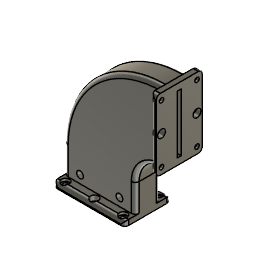
Receiver (Autodesk Fusion 360 design; units mm, degrees)
Autodesk Fusion 360 part; units mm, degrees
sketch "Sketch1" plane through (0, 0, 0) normal (0, 1, 0) x (1, 0, 0)
  circle A0 centre (69, 0) radius 69
  circle A1 centre (69, 0) radius 25
  circle A2 centre (45.471119, -40.686506) radius 22 construction
  line L0 (0, 15) -> (44, 15) construction
  circle A3 centre (37, 15) radius 2.6
  line L1 (22, 15) -> (22, 6) construction
  circle A4 centre (7, 15) radius 2.6
  line L2 (0, 0) -> (0, 25)
  line L3 (0, 25) -> (44, 25)
  line L4 (44, 25) -> (44, 0)
  line L5 (69, -25) -> (69, -69)
  dimension "d1" = 44
  dimension "d2" = 5.2
  dimension "d3" = 15
  dimension "d4" = 25
  dimension "d5" = 50
  dimension "d6" = 10
  constraint coincident L2.start A0
  constraint concentric A0 A1
  constraint tangent A1 A2
  constraint tangent A0 A2
  constraint horizontal L2.start A0.centre
  constraint horizontal L0
  constraint coincident L0 A3.centre
  constraint midpoint L0 L1.start
  constraint perpendicular L0 L1
  constraint symmetric A3 L1 A4
  constraint tangent A0 L2
  constraint perpendicular L0 L2
  constraint perpendicular L2 L3
  constraint perpendicular L3 L4
  constraint coincident L2.start origin
  constraint coincident L4 L0.end
  constraint coincident A1 L4.end
  constraint horizontal A0.centre L4.end
  constraint coincident L0.start L2
  constraint coincident A1 L5.start
  constraint coincident A0 L5.end
  constraint vertical L5
  constraint vertical A0.centre L5.start
  measures "d1" diameter of A2
  measures "d2" diameter of A3
  measures "d3" distance of A3.centre L1
  measures "d4" distance of L2.start L2.end
  measures "d5" diameter of A1
  measures "d6" distance of A3.centre L3
extrude "Extrude1" add sketch "Sketch1" along normal blind 8 contours A0 A1 L3 L4 L5 | A0 L2 L3 picked at (26.77857, -0.136786) picked at (2.261752, 22.293862)
sketch "Sketch2" plane through (0, 8, 0) normal (0, 1, 0) x (-1, 0, 0)
  circle A0 centre (-7, -15) radius 2.6
  circle A1 centre (-37, -15) radius 2.6
  arc A2 (0, 0) -> (-69, 69) centre (-69, 0) ccw
  line L0 (-69, 69) -> (-69, 25)
  arc A3 (-44, 0) -> (-69, 25) centre (-69, 0) ccw
  line L1 (-44, 0) -> (-44, -25)
  line L2 (-44, -25) -> (0, -25)
  line L3 (0, -25) -> (0, 0)
  arc A4 (-49, 0) -> (-74, 19.364917) centre (-69, 0) ccw
  line L4 (-74, 73.830888) -> (-74, 19.364917)
  arc A5 (5, 0) -> (-74, 73.830888) centre (-69, 0) ccw
  line L5 (5, -30) -> (5, 0)
  line L6 (-49, -30) -> (5, -30)
  line L7 (-49, 0) -> (-49, -30)
  line L8 (-69, 20) -> (-74, 20)
  line L9 (-74, 73.830888) -> (-74, 74)
  line L10 (-74, 74) -> (-69, 74)
  line L11 (0, -25) -> (5, -25)
  line L12 (-44, -25) -> (-49, -25)
  line L13 (-69, 69) -> (-69, 74)
  line L14 (-69, 25) -> (-69, 20)
  dimension "d9" = 5
  constraint coincident A4 L8.start
  constraint coincident L4 L8.end
  constraint perpendicular L4 L8
  constraint tangent A4 L8
  constraint parallel L4 L9
  constraint perpendicular L4 L10
  constraint tangent A5 L10
  constraint coincident A5 L10.end
  constraint coincident L2.end L3.start
  constraint coincident L5 L11.end
  constraint perpendicular L5 L11
  constraint coincident L1.end L2.start
  constraint coincident L7 L12.end
  constraint perpendicular L7 L12
  constraint coincident L0.end A3.end
  constraint coincident A2.end L0.start
extrude "Extrude2" add sketch "Sketch2" against normal blind 9.5 contours A2 L3 A5 L5 L11 L13 | A3 L1 A4 L7 L12 L14 picked at (1.666667, -8.333333) picked at (-45.666667, -16.666667)
sketch "Sketch3" plane through (0, 0, -25) normal (0, 0, -1) x (1, 0, 0)
  line L0 (44, 0) -> (0, 0)
  line L1 (0, 0) -> (0, 1.5)
  line L2 (0, 1.5) -> (-5, 1.5)
  line L3 (-5, 1.5) -> (-5, -8)
  line L4 (-5, -8) -> (49, -8)
  line L5 (49, -8) -> (49, 1.5)
  line L6 (49, 1.5) -> (44, 1.5)
  line L7 (44, 1.5) -> (44, 0)
  line L8 (49, -8) -> (49, -16)
  line L9 (49, -16) -> (-5, -16)
  line L10 (-5, -16) -> (-5, -8)
  line L11 (22, -16) -> (22, -8) construction
  line L12 (22, -12) -> (49, -12) construction
  circle A0 centre (44, -12) radius 3
  circle A1 centre (44, -12) radius 1.7
  circle A2 centre (0, -12) radius 3
  circle A3 centre (0, -12) radius 1.7
  circle A4 centre (22, -12) radius 3
  dimension "d12" = 8
  dimension "d13" = 6
  dimension "d14" = 3.4
  dimension "d15" = 5
  dimension "d16" = 6
  constraint coincident L4.end L5.start
  constraint perpendicular L4 L8
  constraint perpendicular L8 L9
  constraint coincident L3.end L4.start
  constraint perpendicular L9 L10
  constraint midpoint L9 L11.start
  constraint midpoint L4 L11.end
  constraint midpoint L11 L12.start
  constraint midpoint L8 L12.end
  constraint coincident L12 A0.centre
  constraint concentric A0 A1
  constraint symmetric L11 A0 A2
  constraint symmetric L11 A1 A3
  constraint coincident L12.start A4.centre
  measures "d12" distance of L4.end L8.end
  measures "d13" diameter of A0
  measures "d14" diameter of A1
  measures "d15" distance of L8 A0.centre
  measures "d16" diameter of A4
sketch "Sketch5" plane through (69, 0, 0) normal (1, 0, 0) x (0, 1, 0)
  line L0 (0, 69) -> (0, 25)
  line L1 (0, 25) -> (-1.5, 25)
  line L2 (-1.5, 25) -> (-1.5, 20)
  line L3 (-1.5, 20) -> (8, 20)
  line L4 (8, 20) -> (8, 74)
  line L5 (8, 74) -> (-1.5, 74)
  line L6 (-1.5, 74) -> (-1.5, 69)
  line L7 (-1.5, 69) -> (0, 69)
  line L8 (16, 74) -> (16, 20)
  line L9 (8, 20) -> (8, 74)
  line L10 (8, 47) -> (16, 47) construction
  line L11 (16, 20) -> (8, 20)
  circle A0 centre (12, 69) radius 3
  line L12 (12, 47) -> (12, 20) construction
  line L13 (8, 74) -> (16, 74)
  circle A1 centre (12, 25) radius 1.7
  circle A2 centre (12, 69) radius 1.7
  circle A3 centre (12, 47) radius 3
  circle A4 centre (12, 25) radius 3
  dimension "d52" = 8
  dimension "d53" = 6
  dimension "d54" = 3.4
  dimension "d55" = 5
  dimension "d56" = 6
  constraint coincident L8.end L11.start
  constraint perpendicular L8 L11
  constraint perpendicular L9 L11
  constraint coincident L8.start L13.end
  constraint perpendicular L9 L13
  constraint midpoint L10.start L9
  constraint midpoint L10.end L8
  constraint midpoint L12.start L10
  constraint midpoint L12.end L11
  constraint coincident A1.centre L12
  constraint concentric A1 A4
  constraint symmetric L10 A0 A4
  constraint symmetric L10 A1 A2
  constraint coincident L12.start A3.centre
  constraint vertical L12
  constraint coincident L4.end L5.start
  measures "d52" distance of L8.end L3.end
  measures "d53" diameter of A4
  measures "d54" diameter of A1
  measures "d55" distance of A1.centre L11
  measures "d56" diameter of A3
extrude "Extrude3" add sketch "Sketch3" against normal blind 4 contours L4 L8 L9 L10 | A0 | A2 picked at (-4.333333, -12) picked at (46.549168, -12.2335) picked at (2.549168, -12.2335)
extrude "Extrude6" add sketch "Sketch5" along normal blind 4 contours L0 L1 L2 L3 L4 L5 L6 L7 L9 | L4 L8 L9 L11 L13 | A0 | A4 picked at (5.333333, 39.666667) picked at (12.07473, 20.669463) picked at (14.398033, 68.104333) picked at (14.555497, 24.850958)
extrude "Extrude4" cut sketch "Sketch3" along normal blind 2 from surface at -4 contours A0 | A2 picked at (46.549168, -12.2335) picked at (2.549168, -12.2335)
extrude "Extrude7" cut sketch "Sketch5" along normal blind 2 contours A0 | A4 picked at (14.398033, 68.104333) picked at (14.555497, 24.850958)
mirror "Mirror1" about plane through (69, -1.5, 25) normal (0, -1, 0) of bodies 1 merged
fillet "Fillet1" radius 3 20 edges at (-5, -11, -10.5) (16.674098, -11, 52.325902) (-5, 8, -10.5) (16.674098, 8, 52.325902) (49, -19, -23) (-5, -19, -23) (22, -19, -21) (49, 16, -23) (22, 16, -21) (-5, 16, -23) (49, 8, -10.5) (54.857864, 8, 14.142136) (49, -11, -10.5) (54.857864, -11, 14.142136) (69, 16, 47) (69, -19, 47) (71, -19, 74) (71, 16, 74) (71, 16, 20) (71, -19, 20)
chamfer "Chamfer1" [suppressed]
sketch "Sketch4" plane through (0, 0, -25) normal (0, 0, -1) x (1, 0, 0)
  circle A0 centre (22, 15) radius 3
  circle A1 centre (0, 15) radius 1.7
  circle A2 centre (44, 15) radius 1.7
  circle A3 centre (44, -12) radius 1.7
  circle A4 centre (0, -12) radius 1.7
  circle A5 centre (22, -12) radius 3
  line L0 (0, 0) -> (0, 3)
  line L1 (0, 3) -> (44, 3)
  line L2 (44, 3) -> (44, 0)
  line L3 (44, 0) -> (0, 0)
  arc A6 (46, -16) -> (49, -13) centre (46, -13) ccw
  line L4 (49, -13) -> (49, 16)
  arc A7 (49, 16) -> (46, 19) centre (46, 16) ccw
  line L5 (46, 19) -> (-2, 19)
  arc A8 (-2, 19) -> (-5, 16) centre (-2, 16) ccw
  line L6 (-5, 16) -> (-5, -13)
  arc A9 (-5, -13) -> (-2, -16) centre (-2, -13) ccw
  line L7 (-2, -16) -> (46, -16)
  circle A10 centre (0, 15) radius 1.3
  circle A11 centre (44, 15) radius 1.3
  circle A12 centre (0, -12) radius 1.3
  circle A13 centre (44, -12) radius 1.3
  dimension "d29" = -0.4
  dimension "d30" = -0.4
  dimension "d31" = -0.4
  dimension "d32" = -0.4
extrude "Extrude5" [suppressed]
fillet "Fillet2" [suppressed]
chamfer "Chamfer2" [suppressed]
sketch "Sketch1 (2)" plane through (0, 0, 0) normal (0, -1, 0) x (1, 0, 0) in component "Plunger"
  circle A0 centre (7, -15) radius 2.6
  circle A1 centre (37, -15) radius 2.6
  arc A2 (69, 69) -> (0, 0) centre (69, 0) ccw
  line L0 (0, 0) -> (0, -25)
  line L1 (0, -25) -> (44, -25)
  line L2 (44, -25) -> (44, 0)
  arc A3 (69, 25) -> (44, 0) centre (69, 0) ccw
  line L3 (69, 25) -> (69, 69)
  line L4 (43, -24) -> (43, 0)
  arc A4 (68, 25.980762) -> (43, 0) centre (69, 0) ccw
  line L5 (68, 25.980762) -> (68, 67.992647)
  arc A5 (68, 67.992647) -> (1, 0) centre (69, 0) ccw
  line L6 (1, 0) -> (1, -24)
  line L7 (1, -24) -> (43, -24)
  circle A6 centre (22, 0) radius 21
  circle A7 centre (22, -34.497692) radius 22
  circle A8 centre (7, -15) radius 3.6
  circle A9 centre (37, -15) radius 3.6
  line L8 (39.636326, -11.4) -> (37, -11.4)
  line L9 (33.4, -15.681741) -> (33.4, -15)
  line L10 (10.6, -15.681741) -> (10.6, -15)
  line L11 (4.363674, -11.4) -> (7, -11.4)
  line L12 (69, 67.992647) -> (68, 67.992647)
  line L13 (69, 25.980762) -> (68, 25.980762)
  line L14 (73, 73) -> (69, 73)
  line L15 (69, 73) -> (69, 69)
  line L16 (73, 21) -> (69, 21)
  line L17 (69, 21) -> (69, 25)
  line L18 (73, 73) -> (73, 21)
  dimension "d37" = 44
  dimension "d38" = 1
  dimension "d39" = 1
  dimension "d43" = 4
  dimension "d44" = 4
  dimension "d45" = 4
  constraint coincident L4.end A6
  constraint tangent L4 A6
  constraint coincident A5.end A6
  constraint coincident A9 L8.end
  constraint tangent A9 L8
  constraint coincident A9 L9.end
  constraint tangent A9 L9
  constraint coincident A8 L10.end
  constraint tangent A8 L10
  constraint coincident A8 L11.end
  constraint tangent A8 L11
  constraint horizontal L11
  constraint vertical L10
  constraint vertical L9
  constraint horizontal L8
  constraint perpendicular L3 L13
  constraint perpendicular L3 L12
  constraint horizontal L14
  constraint coincident A2.start L3.end
  constraint concentric A3 A4
  constraint concentric A2 A5
  constraint tangent L4 A4
  constraint tangent A5 L6
  constraint coincident A3.start L3.start
  constraint perpendicular L16 L17
  constraint perpendicular L16 L18
  constraint perpendicular L14 L15
  constraint vertical L17
  measures "d37" diameter of A7
  measures "d43" distance of L14.start L14.end
  measures "d44" distance of A2.start L14.end
  measures "d45" distance of L16.end A3.start
extrude "Extrude1'" [suppressed] in component "Plunger"
extrude "Extrude2'" [suppressed] in component "Plunger"
component "PogReceiverNew v4" placed x (1, 0, 0) y (0, 1, 0) z (0, 0, 1) at (0, 0, 0)
